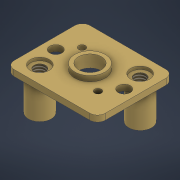
# Autodesk Inventor part: Chapa Superior
Saved by Autodesk Inventor 2021 (Build 250183000, 183)
## iProperties
Created: 2021-01-17
Part Number: Chapa Superior
Material: Genérico
Document SubType Name: Modeling
Designer: João
Density: 1 g/cm^3
Appearance: Padrão
Author: João
Autodesk Inventor part; units mm, degrees
ref_plane "YZ Plane" through (0, 0, 0) normal (1, 0, 0) x (0, 1, 0)
ref_plane "XZ Plane" through (0, 0, 0) normal (0, 1, 0) x (-1, 0, 0)
ref_plane "XY Plane" through (0, 0, 0) normal (0, 0, 1) x (1, 0, 0)
sketch "Esboço1" plane through (0, 0, 0) normal (0, 1, 0) x (-1, 0, 0)
  line L0 (6, 5) -> (-6, 5)
  line L1 (-6, 5) -> (-6, -5)
  line L2 (-6, -5) -> (6, -5)
  line L3 (6, -5) -> (6, 5)
  line L4 (6, 5) -> (-6, -5) construction
  line L5 (-6, 5) -> (6, -5) construction
  point P0 (0, 0)
  dimension "d0" = 12
  dimension "d1" = 10
  constraints: 12 end point, 2 midpoint, 2 parallel, 1 horizontal, 1 perpendicular
  measures "d0" distance of L2.end L1.end
  measures "d1" distance of L1.end L0.end
extrude "Extrusão1" add sketch "Esboço1" along normal blind 0.8
fillet "Arredondamento1" radius 1 4 edges at (-6, 0.4, 5) (6, 0.4, 5) (6, 0.4, -5) (-6, 0.4, -5)
sketch "Esboço2" plane through (0, 0.8, 0) normal (0, 1, 0) x (1, 0, 0)
  circle A0 centre (0, 0) radius 2
  circle A1 centre (0, 0) radius 1.5
  dimension "d5" = 4
  dimension "d6" = 3
  constraints: 2 centre point, 2 coincident
  measures "d5" diameter of A0
  measures "d6" diameter of A1
extrude "Extrusão2" add sketch "Esboço2" along normal blind 0.7
extrude "Extrusão3" cut sketch "Esboço2" against normal blind 0.8 contours A1
sketch "Esboço3" plane through (0, 0.8, 0) normal (0, 1, 0) x (1, 0, 0)
  circle A0 centre (4.5, 0) radius 0.8
  circle A1 centre (0, 0) radius 1.5 projected
  line L0 (0, -1.5) -> (0, 1.5)
  circle A2 centre (-4.5, 0) radius 0.8
  circle A3 centre (0, 0) radius 1.5
  dimension "d11" = 1.6
  constraints: 3 centre point, 2 end point, 2 point on circle, 1 symmetric about line, 1 vertical, 2 other
  measures "d11" diameter of A0
extrude "Extrusão4" cut sketch "Esboço3" against normal blind 0.8 contours A0 | A2
sketch "Esboço4" plane through (0, 0.8, 0) normal (0, 1, 0) x (1, 0, 0)
  circle A0 centre (-3.0146, 1.9633) radius 0.45
  circle A1 centre (0, 0) radius 2 projected
  line L0 (5, 5) -> (-5, 5) projected
  line L1 (-5, -5) -> (5, -5) projected
  circle A2 centre (3.0146, -1.9633) radius 0.45
  dimension "d14" = 0.9
  dimension "d15" = 0.9
  constraints: 2 centre point
  measures "d14" diameter of A0
  measures "d15" diameter of A2
extrude "Extrusão5" cut sketch "Esboço4" against normal blind 0.8 contours A0 | A2
sketch "Esboço5" plane through (0, 0.8, 0) normal (0, 1, 0) x (1, 0, 0)
  circle A0 centre (3.8014, 2.7994) radius 1.25
  circle A1 centre (-3.8014, -2.7994) radius 1.25
  circle A2 centre (3.8014, 2.7994) radius 0.75
  circle A3 centre (-3.8014, -2.7994) radius 0.75
  point P0 (0, 0)
  dimension "d18" = 2.5
  dimension "d19" = 2.5
  dimension "d22" = 1.5
  dimension "d30" = 1.5
  constraints: 4 centre point, 2 coincident
  measures "d18" diameter of A0
  measures "d19" diameter of A1
  measures "d22" diameter of A2
  measures "d30" diameter of A3
extrude "Extrusão6" cut sketch "Esboço5" against normal blind 0.4 contours A0 | A1 | A2 | A3
extrude "Extrusão7" cut sketch "Esboço5" against normal blind 10 contours A2 | A3
sketch "Esboço6" plane through (0, 0, 0) normal (0, -1, 0) x (1, 0, 0)
  circle A0 centre (-3.8014, 2.7994) radius 0.75 projected
  circle A1 centre (-3.8014, 2.7994) radius 1.5
  circle A2 centre (3.8014, -2.7994) radius 0.75 projected
  circle A3 centre (3.8014, -2.7994) radius 1.5
  point P0 (0, 0)
  dimension "d26" = 3
  dimension "d27" = 3
  constraints: 2 centre point, 2 coincident
  measures "d26" diameter of A1
  measures "d27" diameter of A3
extrude "Extrusão8" add sketch "Esboço6" along normal blind 4.6
thread "Rosca1" size "M1.6x0.35" class "6H" standard "ANSI Metric M Profile" full length
thread "Rosca2" size "M1.6x0.35" class "6H" standard "ANSI Metric M Profile" full length
sketch "Esboço10" plane through (0, 0, 0) normal (0, -1, 0) x (1, 0, 0)
  circle A0 centre (0, 0) radius 2 projected
  circle A1 centre (0, 0) radius 1.5 projected
extrude "Extrusão9" add sketch "Esboço10" along normal blind 0.1
